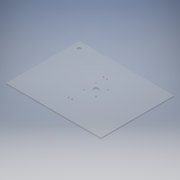
# Autodesk Inventor part: Plaque support
Saved by Autodesk Inventor 2017 (Build 210142000, 142)
## iProperties
Company: FABLAB Frenchmakers
Part Number: Plaque support
Project: 1400-PopCorn Machine
Material: Plastique PMMA
Catalog Web Link: http://www.frenchmakers.com/
Document SubType Name: Modeling
Designer: FABLAB Frenchmakers
Density: 1.188 g/cm^3
Appearance: Polycarbonate - Transparent
Stock Number: 1400-04-05
Mass: 718.603 g
Surface Area: 2499.42 cm^2
Volume: 604.885 cm^3
Author: Adrien MARY
Autodesk Inventor part; units mm, degrees
ref_plane "YZ Plane" through (0, 0, 0) normal (1, 0, 0) x (0, 1, 0)
ref_plane "XZ Plane" through (0, 0, 0) normal (0, 1, 0) x (-1, 0, 0)
ref_plane "XY Plane" through (0, 0, 0) normal (0, 0, 1) x (1, 0, 0)
sketch "Esquisse1" plane through (0, 0, 0) normal (0, 0, 1) x (1, 0, 0)
  line L0 (-198.5, -153) -> (198.5, -153)
  line L1 (198.5, -153) -> (198.5, 153)
  line L2 (198.5, 153) -> (-198.5, 153)
  line L3 (-198.5, 153) -> (-198.5, -153)
  line L4 (-198.5, -153) -> (198.5, 153) construction
  line L5 (198.5, -153) -> (-198.5, 153) construction
  point P0 (0, 0)
  dimension "Largueur_plaque_support" = 397
  dimension "Profondeur_plaque_support" = 306
  constraints: 12 end point, 2 midpoint, 2 parallel, 1 horizontal, 1 perpendicular
  measures "Largueur_plaque_support" distance of L2.end L1.end
  measures "Profondeur_plaque_support" distance of L1.end L0.end
extrude "Embase" add sketch "Esquisse1" along normal mid plane 5
sketch "Trous moteur" plane through (0, 0, 2.5) normal (0, 0, 1) x (1, 0, 0)
  line L0 (-12.4135, -12.4135) -> (37.5865, 37.5865) construction
  line L1 (-12.4135, 37.5865) -> (37.5865, -12.4135) construction
  point P0 (0, 0)
  point P1 (12.5865, 12.5865)
  dimension "Entraxe_vis_moteur" = 50
  dimension "d5" = 50
  dimension "Entraxe_engrenage" = 17.8
  constraints: 4 coincident, 4 end point, 2 horizontal alignment, 2 midpoint, 2 vertical alignment, 1 point on line
  measures "Entraxe_vis_moteur" distance of L1.start L0.end
  measures "d5" distance of L0.end L1.end
  measures "Entraxe_engrenage" distance from line of point (0, 0) L1
hole "Passage vis moteur" at (-12.4135, 37.5865, 2.5) at (37.5865, 37.5865, 2.5) at (37.5865, -12.4135, 2.5) at (-12.4135, -12.4135, 2.5) direction (0, 0, -1) diameter 4.5 end through all clearance for "Vis à tête plate fraisée ISO 2009/7046" size "M4" standard "ISO"
hole "Passage axe moteur" at (12.5865, 12.5865, 2.5) direction (0, 0, -1) diameter 21 end through all
sketch "Esquisse3" plane through (0, 0, 2.5) normal (0, 0, 1) x (1, 0, 0)
  point P0 (0, 0)
  point P1 (-16.5, 73.3)
  point P2 (-1.5, 73.3)
  dimension "Entraxe_fication" = 15
  dimension "Demi_entraxe" = 73.3
  dimension "Décalage" = 1.5
  constraints: 1 horizontal alignment
  measures "Entraxe_fication" distance of point (-1.5, 73.3) point (-16.5, 73.3)
  measures "Demi_entraxe" vertical distance of point (0, 0) point (-16.5, 73.3)
  measures "Décalage" horizontal distance of point (0, 0) point (-1.5, 73.3)
hole "Passage vis bras" at (-16.5, 73.3, 2.5) at (-1.5, 73.3, 2.5) direction (0, 0, -1) diameter 5.5 end through all clearance for "Vis à tête plate fraisée ISO 2009/7046" size "M5" standard "ISO"
mirror "Symétrie passage vis bras" about plane through (0, 0, 0) normal (0, 1, 0) of "Passage vis bras"
sketch "Esquisse4" plane through (0, 0, 2.5) normal (0, 0, 1) x (1, 0, 0)
  point P0 (0, 0)
  point P1 (-170, 125)
  dimension "d31" = 170
  dimension "d32" = 125
  measures "d31" horizontal distance of point (0, 0) point (-170, 125)
  measures "d32" vertical distance of point (0, 0) point (-170, 125)
hole "Perçage4" at (-170, 125, 2.5) direction (0, 0, -1) diameter 15 end through all
equation "\"d5\" = Entraxe_vis_moteur"
